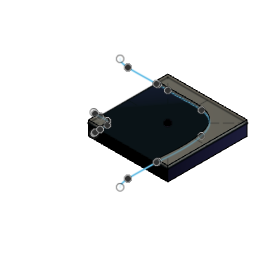
Turn (Autodesk Fusion 360 design; units mm, degrees)
Autodesk Fusion 360 part; units mm, degrees
sketch "Sketch1" plane through (0, 0, 0) normal (0, 1, 0) x (1, 0, 0)
  line L0 (3.5, -3.5) -> (-3.5, -3.5)
  line L1 (-3.5, -3.5) -> (-3.5, 3.5)
  line L2 (-3.5, 3.5) -> (3.5, 3.5)
  line L3 (3.5, 3.5) -> (3.5, -3.5)
  line L4 (3.5, -3.5) -> (-3.5, 3.5) construction
  line L5 (-3.5, -3.5) -> (3.5, 3.5) construction
  line L6 (-3.5, 0) -> (3.5, 0) construction
  line L7 (0, 3.5) -> (0, -3.5) construction
  spline S0 degree 5 poles (-2.4495, -4.0862) (-2.4531, -4.0821) (-2.4598, -4.073) (-2.4693, -4.0564) (-2.4806, -4.0283) (-2.4922, -3.9831) (-2.5012, -3.9279) (-2.5076, -3.8624) (-2.5108, -3.7868) (-2.5105, -3.701) (-2.5067, -3.6054) (-2.4998, -3.501) (-2.4909, -3.3892) (-2.482, -3.2726) (-2.4758, -3.1541) (-2.4754, -3.0372) (-2.4839, -2.9253) (-2.5041, -2.8219) (-2.538, -2.7297) (-2.5868, -2.6509) (-2.6509, -2.5868) (-2.7297, -2.538) (-2.8219, -2.5041) (-2.9253, -2.4839) (-3.0372, -2.4754) (-3.1541, -2.4758) (-3.2726, -2.482) (-3.3892, -2.4909) (-3.501, -2.4998) (-3.6054, -2.5067) (-3.701, -2.5105) (-3.7868, -2.5108) (-3.8624, -2.5076) (-3.9279, -2.5012) (-3.9831, -2.4922) (-4.0283, -2.4806) (-4.0564, -2.4693) (-4.073, -2.4599) (-4.0821, -2.4531) (-4.0862, -2.4495) knots 0 0 0 0 0 0 0.028571 0.057143 0.085714 0.114286 0.142857 0.171429 0.2 0.228571 0.257143 0.285714 0.314286 0.342857 0.371429 0.4 0.428571 0.457143 0.485714 0.514286 0.542857 0.571429 0.6 0.628571 0.657143 0.685714 0.714286 0.742857 0.771429 0.8 0.828571 0.857143 0.885714 0.914286 0.942857 0.971429 1 1 1 1 1 1
  spline S1 degree 5 poles (-3.5, 2.5003) (-3.592, 2.5004) (-3.7772, 2.4999) (-4.0588, 2.4968) (-4.4399, 2.4888) (-4.9136, 2.4773) (-5.3682, 2.4705) (-5.787, 2.4753) (-6.1548, 2.4975) (-6.4627, 2.5408) (-6.7098, 2.6058) (-6.8605, 2.6746) (-6.9484, 2.7352) (-6.9959, 2.7796) (-7.017, 2.8028) knots 0 0 0 0 0 0 0.1 0.2 0.3 0.4 0.5 0.6 0.7 0.8 0.9 1 1 1 1 1 1
  line L8 (-3.1261, 2.4997) -> (-3.8739, 2.5008)
  spline S2 degree 5 poles (-2.4927, 2.4927) (-2.524, 2.4933) (-2.5888, 2.4946) (-2.6927, 2.4972) (-2.8416, 2.5014) (-3.0292, 2.5069) (-3.199, 2.5113) (-3.3329, 2.5134) (-3.4194, 2.5126) (-3.4604, 2.5092) (-3.4728, 2.5048) (-3.4769, 2.5018) (-3.4853, 2.5005) (-3.4945, 2.5003) (-3.5, 2.5003) knots 0 0 0 0 0 0 0.1 0.2 0.3 0.4 0.5 0.6 0.7 0.8 0.9 1 1 1 1 1 1
  line L9 (-2.391, 2.4907) -> (-2.5943, 2.4946)
  line L10 (-3.398, 2.5001) -> (-3.602, 2.5004)
  spline S3 degree 5 poles (2.8028, -7.0169) (2.7796, -6.9959) (2.7352, -6.9484) (2.6746, -6.8605) (2.6058, -6.7098) (2.5409, -6.4627) (2.4975, -6.1548) (2.4753, -5.787) (2.4705, -5.3682) (2.4773, -4.9135) (2.4888, -4.4399) (2.4968, -4.0588) (2.4999, -3.7772) (2.5004, -3.592) (2.5003, -3.5) knots 0 0 0 0 0 0 0.1 0.2 0.3 0.4 0.5 0.6 0.7 0.8 0.9 1 1 1 1 1 1
  line L11 (2.5009, -3.8739) -> (2.4997, -3.1261)
  spline S4 degree 5 poles (2.5003, -3.5) (2.5003, -3.4902) (2.5001, -3.4756) (2.4995, -3.4685) (2.5012, -3.4612) (2.5205, -3.3295) (2.5597, -2.9945) (2.6072, -2.4508) (2.6438, -1.7375) (2.6461, -0.9259) (2.5908, -0.0993) (2.4593, 0.6617) (2.2418, 1.2985) (1.941, 1.7877) (1.5675, 2.1302) (1.137, 2.345) (0.6663, 2.4609) (0.1707, 2.5098) (-0.3399, 2.5187) (-0.8612, 2.5083) (-1.3923, 2.4938) (-1.8259, 2.4871) (-2.1569, 2.4876) (-2.3803, 2.4905) (-2.4927, 2.4927) knots 0 0 0 0 0 0 0.05 0.1 0.15 0.2 0.25 0.3 0.35 0.4 0.45 0.5 0.55 0.6 0.65 0.7 0.75 0.8 0.85 0.9 0.95 1 1 1 1 1 1
  line L12 (2.5018, -4.529) -> (2.4988, -2.471)
  line L13 (-1.3885, 2.4716) -> (-3.5969, 2.5138)
  point P0 (-2.5013, -3.9197)
  point P1 (-2.4979, -3.4799)
  point P2 (-2.5053, -2.8327)
  point P3 (-2.8327, -2.5053)
  point P4 (-3.4799, -2.4979)
  point P5 (-3.9197, -2.5013)
  point P6 (2.4925, -6.018)
  point P7 (2.5126, -3.3792)
  point P8 (2.468, 0.5041)
  point P9 (0.5041, 2.468)
  point P10 (-3.3793, 2.5126)
  point P11 (-6.018, 2.4924)
  dimension "d1" = 0
  dimension "d2" = 0
  constraint horizontal L0
  constraint perpendicular L0 L1
  constraint parallel L0 L2
  constraint parallel L1 L3
  constraint coincident L4 origin
  constraint coincident L5 origin
  constraint midpoint L1 L6.start
  constraint midpoint L3 L6.end
  constraint midpoint L2 L7.start
  constraint midpoint L0 L7.end
  constraint coincident L4 S2.start
  constraint coincident L1 S1.start
  constraint midpoint S1.start L8
  constraint midpoint S2.start L9
  constraint midpoint S1.start L10
  constraint coincident L0 S3.end
  constraint midpoint S3.end L11
  constraint midpoint S3.end L12
  constraint midpoint S2.start L13
  measures "d1" distance of L1.end L2.end
  measures "d2" distance of L0.end L1.end
sketch "Sketch2" plane through (0, 0, 0) normal (0, 1, 0) x (1, 0, 0)
  line L0 (3.5, 3.5) -> (-3.5, 3.5)
  line L1 (-3.5, 3.5) -> (-3.5, -3.5)
  line L2 (-3.5, -3.5) -> (3.5, -3.5)
  line L3 (3.5, -3.5) -> (3.5, 3.5)
  line L4 (3.5, 3.5) -> (-3.5, -3.5) construction
  line L5 (-3.5, 3.5) -> (3.5, -3.5) construction
  line L6 (2.5, -3.5) -> (2.5, 3.5)
  line L7 (-2.5, 3.5) -> (-2.5, -3.5)
  dimension "d3" = 0
  dimension "d4" = 0
  dimension "d5" = 0
  dimension "d6" = 0
  constraint horizontal L0
  constraint perpendicular L0 L1
  constraint parallel L0 L2
  constraint parallel L1 L3
  constraint coincident L4 origin
  constraint coincident L5 origin
  constraint coincident L2 L6.start
  constraint coincident L0 L6.end
  constraint coincident L0 L7.start
  constraint coincident L2 L7.end
  constraint vertical L7
  constraint vertical L6
  measures "d3" distance of L1.end L2.end
  measures "d4" distance of L0.end L1.end
  measures "d5" distance of L1 L7
  measures "d6" distance of L0.start L6.end
extrude "Extrude2" add sketch "Sketch1" along normal blind 0.25 contours L0 L1 L2 L3 S2 L9 S4 L13 | L0 L1 S0 | L1 S2 L13 makes body 1 at (-3.004, 0, 3.0141) makes body 2 at (-0.0021, 0, -3.1694)
extrude "Extrude3" add sketch "Sketch2" against normal blind 1 separate body makes body 3
equation "d62 = curb_t"
equation "d80 = -tile_t"
equation "tile_t = 1 mm"
equation "curb_t = 0.25 mm"
equation "d1 = tile_size"
equation "d2 = tile_size"
equation "d3 = tile_size"
equation "d4 = tile_size"
equation "d5 = curb_w"
equation "d6 = curb_w"
